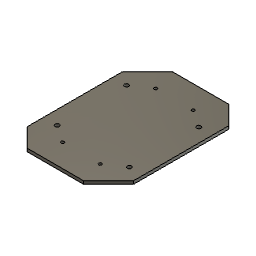
Cube Holder (Autodesk Fusion 360 design; units mm, degrees)
Autodesk Fusion 360 part; units mm, degrees
sketch "Sketch1" plane through (0, 0, 0) normal (0, 1, 0) x (1, 0, 0)
  line L0 (17.145, 0) -> (68.58, 0)
  line L1 (91.44, 22.86) -> (91.44, 109.855)
  line L2 (74.295, 127) -> (22.86, 127)
  line L3 (0, 104.14) -> (0, 17.145)
  circle A0 centre (12.7, 31.75) radius 1.905
  circle A1 centre (78.74, 95.25) radius 1.905
  circle A2 centre (78.74, 31.75) radius 1.905
  circle A3 centre (12.7, 95.25) radius 1.905
  circle A4 centre (28.525, 20.96) radius 1.375
  circle A5 centre (62.915, 20.96) radius 1.375
  circle A6 centre (62.915, 106.04) radius 1.375
  circle A7 centre (28.525, 106.04) radius 1.375
  line L4 (22.86, 127) -> (0, 104.14)
  line L5 (91.44, 109.855) -> (74.295, 127)
  line L6 (68.58, 0) -> (91.44, 22.86)
  line L7 (17.145, 0) -> (0, 17.145)
  point P0 (91.44, 0)
  point P1 (91.44, 127)
  point P2 (0, 127)
  dimension "d1" = 91.44
  dimension "d8" = 2.75
  dimension "d63" = 22.86
  dimension "d64" = 22.86
  dimension "d65" = 17.145
  dimension "d66" = 17.145
  dimension "d67" = 22.86
  dimension "d68" = 22.86
  dimension "d69" = 17.145
  dimension "d70" = 17.145
  constraint horizontal L0
  constraint vertical L1
  constraint horizontal L2
  constraint vertical L3
  constraint coincident P2 L2
  constraint coincident P2 L3
  constraint coincident P1 L1
  constraint coincident P1 L2
  constraint coincident P0 L0
  constraint coincident P0 L1
  constraint coincident origin L0
  constraint coincident origin L3
  measures "d1" distance of origin P0
  measures "d8" diameter of A7
  measures "d63" distance of P2 L2.end
  measures "d64" distance of P2 L3.start
  measures "d65" distance of P1 L1.end
  measures "d66" distance of P1 L2.start
  measures "d67" distance of P0 L0.end
  measures "d68" distance of P0 L1.start
  measures "d69" distance of origin L0.start
  measures "d70" distance of origin L3.end
extrude "Extrude5" add sketch "Sketch1" along normal blind 2.794
equation "d64 = d63"
equation "d66 = d65"
equation "d68 = d67"
equation "d70 = d69"
